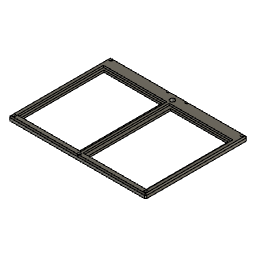
SensorBox-Zanzibar_Waterproofing v12 (Autodesk Fusion 360 design; units mm, degrees)
Autodesk Fusion 360 part; units mm, degrees
note: some values were not read from the file. Set by a fixed rule: which face or edge a step refers to.
sketch "Sketch1" plane through (0, 0, 0) normal (0, 0, 1) x (1, 0, 0) in component "Panel_Top"
  line L0 (27.5294, 43.3117) -> (202.5294, 43.3117)
  line L1 (202.5294, 43.3117) -> (202.5294, 173.3117)
  line L2 (202.5294, 173.3117) -> (27.5294, 173.3117)
  line L3 (27.5294, 173.3117) -> (27.5294, 43.3117)
  line L4 (197.5294, 159.5617) -> (32.5294, 159.5617)
  line L5 (32.5294, 159.5617) -> (32.5294, 49.5617)
  line L6 (32.5294, 49.5617) -> (197.5294, 49.5617)
  line L7 (197.5294, 49.5617) -> (197.5294, 159.5617)
  line L8 (197.5294, 159.5617) -> (32.5294, 49.5617) construction
  line L9 (32.5294, 159.5617) -> (197.5294, 49.5617) construction
  line L10 (116.5294, 159.5617) -> (113.5294, 159.5617)
  line L11 (113.5294, 159.5617) -> (113.5294, 49.5617)
  line L12 (113.5294, 49.5617) -> (116.5294, 49.5617)
  line L13 (116.5294, 49.5617) -> (116.5294, 159.5617)
  line L14 (116.5294, 159.5617) -> (113.5294, 49.5617) construction
  line L15 (113.5294, 159.5617) -> (116.5294, 49.5617) construction
  line L16 (27.5294, 108.3117) -> (32.5294, 104.5617)
  line L17 (115.0294, 43.3117) -> (115.0294, 49.5617)
  line L18 (109.5294, 157.0617) -> (35.5294, 157.0617)
  line L19 (35.5294, 157.0617) -> (35.5294, 52.0617)
  line L20 (35.5294, 52.0617) -> (109.5294, 52.0617)
  line L21 (109.5294, 52.0617) -> (109.5294, 157.0617)
  line L22 (120.5294, 157.0617) -> (194.5294, 157.0617)
  line L23 (194.5294, 157.0617) -> (194.5294, 52.0617)
  line L24 (194.5294, 52.0617) -> (120.5294, 52.0617)
  line L25 (120.5294, 52.0617) -> (120.5294, 157.0617)
  circle A0 centre (115, 165) radius 3
  circle A1 centre (30.9, 47.1432) radius 1
  line L26 (115.0294, 120.0286) -> (115.0294, 79)
  circle A2 centre (199.1589, 47.1432) radius 1
  circle A3 centre (31.1445, 170.3984) radius 1
  circle A4 centre (198.9143, 170.3984) radius 1
  circle A5 centre (115.0294, 46.0617) radius 1
  line L27 (115.0294, 45.0617) -> (115.0294, 43.3117)
  line L28 (115.0294, 45.0617) -> (115.0294, 43.3117)
  circle A6 centre (31.1445, 170.3984) radius 2
  circle A7 centre (30.9, 47.1432) radius 2
  circle A8 centre (115.0294, 46.0617) radius 2
  circle A9 centre (199.1589, 47.1432) radius 2
  circle A10 centre (198.9143, 170.3984) radius 2
  circle A11 centre (103.0229, 171.842) radius 1
  circle A12 centre (127.025, 171.7921) radius 1
  circle A13 centre (103.0229, 171.842) radius 2
  circle A14 centre (127.025, 171.7921) radius 2
  point P0 (115.0294, 104.5617)
  point P1 (115.0294, 104.5617)
  point P2 (73.0294, 104.5617)
  point P3 (115, 165)
  point P4 (103.0229, 171.842)
  dimension "d29" = 175
  dimension "d30" = 130
  dimension "d31" = 165
  dimension "d32" = 110
  dimension "d33" = 3
  dimension "d34" = 81
  dimension "d35" = 81
  dimension "d36" = 74
  dimension "d37" = 105
  dimension "d38" = 74
  dimension "d39" = 105
  dimension "d47" = 6
  dimension "d85" = 2
  dimension "d86" = 2
  dimension "d89" = 2
  dimension "d90" = 2
  dimension "d92" = 2
  dimension "d93" = 1.75
  dimension "d213" = 4
  dimension "d214" = 4
  dimension "d215" = 4
  dimension "d216" = 4
  dimension "d217" = 4
  dimension "d223" = 2
  dimension "d224" = 2
  dimension "d225" = 4
  dimension "d226" = 4
  constraint horizontal L0
  constraint vertical L1
  constraint horizontal L2
  constraint vertical L3
  constraint horizontal L4
  constraint perpendicular L4 L5
  constraint parallel L4 L6
  constraint parallel L5 L7
  constraint coincident L8 P1
  constraint coincident L9 P1
  constraint horizontal L10
  constraint perpendicular L10 L11
  constraint parallel L10 L12
  constraint parallel L11 L13
  constraint coincident L14 P1
  constraint coincident L15 P1
  constraint coincident P1 P0
  constraint midpoint L3 L16.start
  constraint midpoint L5 L16.end
  constraint midpoint L0 L17.start
  constraint midpoint L6 L17.end
  constraint perpendicular L6 L17
  constraint equal L16 L17
  constraint horizontal L18
  constraint perpendicular L18 L19
  constraint parallel L18 L20
  constraint parallel L19 L21
  constraint perpendicular L22 L23
  constraint parallel L22 L24
  constraint parallel L23 L25
  constraint parallel L25 L26
  constraint coincident L17 A5.centre
  constraint coincident A5 L27.start
  constraint coincident L17 L27.start
  constraint perpendicular L0 L27
  constraint coincident P3 A0.centre
  constraint concentric A3 A6
  constraint concentric A1 A7
  constraint concentric A5 A8
  constraint concentric A2 A9
  constraint concentric A4 A10
  constraint coincident P4 A11.centre
  constraint concentric A11 A13
  constraint concentric A12 A14
  measures "d29" distance of L0.start L0.end
  measures "d30" distance of L0.start L2.end
  measures "d31" distance of L5.end L6.end
  measures "d32" distance of L4.end L5.end
  measures "d33" distance of L11.end L12.end
  measures "d34" distance of L5.end L11.end
  measures "d35" distance of L6.end L12.end
  measures "d36" distance of L19.end L20.end
  measures "d37" distance of L18.end L19.end
  measures "d38" distance of L23.end L24.end
  measures "d39" distance of L22.end L23.end
  measures "d47" diameter of A0
  measures "d85" diameter of A1
  measures "d86" diameter of A2
  measures "d89" diameter of A3
  measures "d90" diameter of A4
  measures "d92" diameter of A5
  measures "d93" distance of L17.start L27.start
  measures "d213" diameter of A6
  measures "d214" diameter of A7
  measures "d215" diameter of A8
  measures "d216" diameter of A9
  measures "d217" diameter of A10
  measures "d223" diameter of A11
  measures "d224" diameter of A12
  measures "d225" diameter of A13
  measures "d226" diameter of A14
extrude "Extrude2" add sketch "Sketch1" along normal blind 5 contours L0 L3 L5 L6 L12 L16 L17 L27 L28 A8 | L0 L1 L2 L3 L4 L5 L6 L7 L10 L12 L16 L17 L27 L28 A8 A13 A14 | L17 A5 L27 L28 A8 | L17 A5 L27 L28 A8 | L17 A5 | L17 A5 | L2 A13 | L2 A14 | L4 L6 L10 L11 L12 L13 | A0 | A1 | A2 | A3 | A4 | A6 | A7 | A9 | A10 | A11 | A12 picked at (103.0478, 173.1542) picked at (127.0499, 173.1375) makes body 1 in component "Panel_Top"
extrude "Extrude3" add sketch "Sketch1" along normal blind 2.5 contours L4 L5 L6 L11 | L4 L6 L7 L13 bodies 1 in component "Panel_Top"
chamfer "Chamfer1" distance 1.5 angle 45 8 edges at (115.0294, 173.3117, 5) (115.0294, 43.3117, 5) (202.5294, 108.3117, 5) (202.5294, 43.3117, 2.5) (202.5294, 173.3117, 2.5) (27.5294, 173.3117, 2.5) (27.5294, 108.3117, 5) (27.5294, 43.3117, 2.5) on bodies 1 in component "Panel_Top"
extrude "Extrude4" cut sketch "Sketch1" along normal blind 10 contours A0 bodies 1 in component "Panel_Top"
sketch "Sketch1 (2)" plane through (0, 0, 0) normal (0, 0, 1) x (1, 0, 0) in component "Box"
  line L0 (200.9294, 173.7581) -> (25.9294, 173.7581)
  line L1 (200.9294, 43.7581) -> (200.9294, 173.7581)
  line L2 (25.9294, 43.7581) -> (200.9294, 43.7581)
  line L3 (25.9294, 173.7581) -> (25.9294, 43.7581)
  line L4 (100.1921, 43.7581) -> (100.1921, 49.5617)
  line L5 (76.1646, 173.7581) -> (76.1646, 167.0617)
  line L6 (100.1292, 173.7581) -> (100.1292, 167.0617)
  line L7 (195.9294, 170.3581) -> (30.9294, 170.3581)
  line L8 (30.9294, 170.3581) -> (30.9294, 50.3581)
  line L9 (30.9294, 50.3581) -> (195.9294, 50.3581)
  line L10 (195.9294, 50.3581) -> (195.9294, 170.3581)
  line L11 (195.9294, 170.3581) -> (30.9294, 50.3581) construction
  line L12 (30.9294, 170.3581) -> (195.9294, 50.3581) construction
  circle A0 centre (29.5445, 170.3984) radius 1
  line L13 (25.9294, 173.7581) -> (30.9294, 170.3581)
  circle A1 centre (197.5001, 170.373) radius 1
  circle A2 centre (29.3, 47.1432) radius 1
  circle A3 centre (197.5001, 47.1432) radius 1
  circle A4 centre (113.425, 46.5081) radius 1
  line L14 (113.4294, 43.7581) -> (113.4294, 45.5081)
  line L15 (35.5295, 157.0617) -> (191.3258, 157.0617)
  line L16 (191.3258, 157.0617) -> (191.3258, 52.0619)
  line L17 (191.3258, 52.0619) -> (35.5295, 52.0619)
  line L18 (35.5295, 52.0619) -> (35.5295, 157.0617)
  line L19 (99.995, 157.0617) -> (129.995, 157.0617)
  line L20 (129.995, 157.0617) -> (129.995, 169.1149)
  line L21 (129.995, 169.1149) -> (99.995, 169.1149)
  line L22 (99.995, 169.1149) -> (99.995, 157.0617)
  line L23 (35.5295, 135.5381) -> (30.9294, 135.3581)
  line L24 (65.9281, 157.0617) -> (65.9281, 170.6598)
  line L25 (162.4706, 157.0617) -> (162.4706, 168.7581)
  line L26 (191.3258, 133.7581) -> (195.9294, 133.7581)
  line L27 (35.5295, 83.7581) -> (30.9294, 83.7581)
  line L28 (191.3258, 83.7581) -> (195.9294, 83.7581)
  line L29 (67.5294, 52.0619) -> (67.5294, 50.3581)
  line L30 (162.4706, 52.0619) -> (162.4706, 50.3581)
  line L31 (50, 162) -> (80, 162)
  line L32 (80, 162) -> (80, 157)
  line L33 (80, 157) -> (50, 157)
  line L34 (50, 157) -> (50, 162)
  line L35 (180, 162) -> (150, 162)
  line L36 (180, 157) -> (180, 162)
  line L37 (150, 157) -> (180, 157)
  line L38 (150, 162) -> (150, 157)
  line L39 (25.9294, 99.9709) -> (30.9294, 99.9709)
  line L40 (195.9294, 99.9709) -> (200.9294, 99.9709)
  line L41 (159.383, 124.881) -> (70.383, 124.881)
  line L42 (70.383, 124.881) -> (70.383, 150.281)
  line L43 (70.383, 150.281) -> (159.383, 150.281)
  line L44 (159.383, 150.281) -> (159.383, 124.881)
  line L45 (159.383, 124.881) -> (70.383, 150.281) construction
  line L46 (70.383, 124.881) -> (159.383, 150.281) construction
  line L47 (94.9348, 114.6136) -> (54.9348, 114.6136)
  line L48 (54.9348, 114.6136) -> (54.9348, 61.6136)
  line L49 (54.9348, 61.6136) -> (94.9348, 61.6136)
  line L50 (94.9348, 61.6136) -> (94.9348, 114.6136)
  line L51 (94.9348, 114.6136) -> (54.9348, 61.6136) construction
  line L52 (54.9348, 114.6136) -> (94.9348, 61.6136) construction
  line L53 (54.9348, 114.6136) -> (64.9348, 114.6136)
  line L54 (64.9348, 114.6136) -> (64.9348, 104.6136)
  line L55 (64.9348, 104.6136) -> (54.9348, 104.6136)
  line L56 (54.9348, 104.6136) -> (54.9348, 114.6136)
  line L57 (54.9348, 61.6136) -> (64.9348, 61.6136)
  line L58 (64.9348, 61.6136) -> (64.9348, 71.6136)
  line L59 (64.9348, 71.6136) -> (54.9348, 71.6136)
  line L60 (54.9348, 71.6136) -> (54.9348, 61.6136)
  line L61 (94.9348, 114.6136) -> (84.9348, 114.6136)
  line L62 (84.9348, 114.6136) -> (84.9348, 104.6136)
  line L63 (84.9348, 104.6136) -> (94.9348, 104.6136)
  line L64 (94.9348, 104.6136) -> (94.9348, 114.6136)
  line L65 (94.9348, 61.6136) -> (84.9348, 61.6136)
  line L66 (84.9348, 61.6136) -> (84.9348, 71.6136)
  line L67 (84.9348, 71.6136) -> (94.9348, 71.6136)
  line L68 (94.9348, 71.6136) -> (94.9348, 61.6136)
  line L69 (64.9348, 104.6136) -> (51.9348, 104.6136)
  line L70 (51.9348, 104.6136) -> (51.9348, 117.6136)
  line L71 (51.9348, 117.6136) -> (64.9348, 117.6136)
  line L72 (64.9348, 117.6136) -> (64.9348, 104.6136)
  line L73 (64.9348, 71.6136) -> (51.9348, 71.6136)
  line L74 (51.9348, 71.6136) -> (51.9348, 58.6136)
  line L75 (51.9348, 58.6136) -> (64.9348, 58.6136)
  line L76 (64.9348, 58.6136) -> (64.9348, 71.6136)
  line L77 (84.9348, 71.6136) -> (97.9348, 71.6136)
  line L78 (97.9348, 71.6136) -> (97.9348, 58.6136)
  line L79 (97.9348, 58.6136) -> (84.9348, 58.6136)
  line L80 (84.9348, 58.6136) -> (84.9348, 71.6136)
  line L81 (84.9348, 104.6136) -> (97.9348, 104.6136)
  line L82 (97.9348, 104.6136) -> (97.9348, 117.6136)
  line L83 (97.9348, 117.6136) -> (84.9348, 117.6136)
  line L84 (84.9348, 117.6136) -> (84.9348, 104.6136)
  line L85 (159.2809, 101.4464) -> (104.2809, 101.4464)
  line L86 (104.2809, 101.4464) -> (104.2809, 76.4464)
  line L87 (104.2809, 76.4464) -> (159.2809, 76.4464)
  line L88 (159.2809, 76.4464) -> (159.2809, 101.4464)
  line L89 (159.2809, 101.4464) -> (104.2809, 76.4464) construction
  line L90 (104.2809, 101.4464) -> (159.2809, 76.4464) construction
  circle A5 centre (104.2809, 101.4464) radius 1.25
  circle A6 centre (104.2809, 76.4464) radius 1.25
  circle A7 centre (159.2809, 101.4464) radius 1.25
  circle A8 centre (159.2809, 76.4464) radius 1.25
  circle A9 centre (70.383, 150.281) radius 1.6
  circle A10 centre (70.383, 124.881) radius 1.6
  circle A11 centre (159.383, 150.281) radius 1.6
  circle A12 centre (159.383, 124.881) radius 1.6
  line L91 (30.9294, 116.2794) -> (35.5295, 116.2794)
  line L92 (35.5295, 116.2794) -> (35.5295, 101.2775)
  line L93 (35.5295, 101.2775) -> (30.9294, 101.2775)
  line L94 (30.9294, 101.2775) -> (30.9294, 116.2794)
  line L95 (191.3258, 101.2799) -> (195.9294, 101.2799)
  line L96 (195.9294, 101.2799) -> (195.9294, 116.2759)
  line L97 (195.9294, 116.2759) -> (191.3258, 116.2759)
  line L98 (191.3258, 116.2759) -> (191.3258, 101.2799)
  circle A13 centre (104.2809, 101.4464) radius 2.25
  circle A14 centre (104.2809, 76.4464) radius 2.25
  circle A15 centre (159.2809, 101.4464) radius 2.25
  circle A16 centre (159.2809, 76.4464) radius 2.25
  circle A17 centre (127.0246, 171.7917) radius 1
  line L99 (114.995, 172.8091) -> (114.995, 171)
  circle A18 centre (103.0221, 171.8383) radius 1
  point P0 (113.4294, 110.3581)
  point P1 (113.4294, 110.3581)
  point P2 (114.883, 137.581)
  point P3 (74.9348, 88.1136)
  point P4 (113.4294, 110.3581)
  point P5 (131.7809, 88.9464)
  dimension "d50" = 175
  dimension "d51" = 130
  dimension "d68" = 5.8036
  dimension "d69" = 165
  dimension "d70" = 120
  dimension "d77" = 2
  dimension "d82" = 2
  dimension "d83" = 2
  dimension "d84" = 2
  dimension "d94" = 2
  dimension "d95" = 1.75
  dimension "d120" = 30
  dimension "d127" = 35
  dimension "d128" = 35
  dimension "d146" = 89
  dimension "d147" = 25.4
  dimension "d155" = 40
  dimension "d156" = 53
  dimension "d157" = 10
  dimension "d158" = 10
  dimension "d159" = 10
  dimension "d160" = 10
  dimension "d161" = 10
  dimension "d162" = 10
  dimension "d163" = 10
  dimension "d164" = 10
  dimension "d165" = 13
  dimension "d166" = 13
  dimension "d167" = 13
  dimension "d168" = 13
  dimension "d169" = 13
  dimension "d170" = 13
  dimension "d171" = 13
  dimension "d172" = 13
  dimension "d175" = 55
  dimension "d176" = 25
  dimension "d177" = 2.5
  dimension "d178" = 2.5
  dimension "d179" = 2.5
  dimension "d180" = 2.5
  dimension "d181" = 3.2
  dimension "d182" = 3.2
  dimension "d183" = 3.2
  dimension "d184" = 3.2
  dimension "d207" = 4.5
  dimension "d208" = 4.5
  dimension "d209" = 4.5
  dimension "d210" = 4.5
  dimension "d221" = 2
  dimension "d222" = 2
  constraint horizontal L2
  constraint vertical L1
  constraint horizontal L0
  constraint vertical L3
  constraint coincident L2 L4.start
  constraint coincident L0 L5.start
  constraint coincident L0 L6.start
  constraint horizontal L7
  constraint perpendicular L7 L8
  constraint parallel L7 L9
  constraint parallel L8 L10
  constraint coincident L11 P4
  constraint coincident L12 P4
  constraint midpoint L2 L14.start
  constraint coincident A4 L14.end
  constraint perpendicular L2 L14
  constraint horizontal L15
  constraint vertical L16
  constraint horizontal L17
  constraint vertical L18
  constraint horizontal L19
  constraint vertical L20
  constraint horizontal L21
  constraint vertical L22
  constraint coincident L15 L19.start
  constraint coincident L8 L23.end
  constraint coincident L18 L23.start
  constraint coincident L15 L24.start
  constraint perpendicular L7 L24
  constraint coincident L10 L28.end
  constraint perpendicular L10 L28
  constraint coincident L16 L28.start
  constraint coincident L10 L26.end
  constraint perpendicular L10 L26
  constraint coincident L16 L26.start
  constraint coincident L17 L29.start
  constraint coincident L9 L29.end
  constraint perpendicular L9 L29
  constraint coincident L17 L30.start
  constraint coincident L9 L30.end
  constraint perpendicular L9 L30
  constraint horizontal L31
  constraint vertical L32
  constraint horizontal L33
  constraint vertical L34
  constraint coincident P4 P1
  constraint equal L23 L26
  constraint coincident L8 L27.end
  constraint perpendicular L8 L27
  constraint coincident L3 L39.start
  constraint coincident L8 L39.end
  constraint perpendicular L8 L39
  constraint coincident L10 L40.start
  constraint coincident L1 L40.end
  constraint perpendicular L1 L40
  constraint equal L39 L40
  constraint horizontal L41
  constraint perpendicular L41 L42
  constraint parallel L41 L43
  constraint parallel L42 L44
  constraint coincident L45 P2
  constraint coincident L46 P2
  constraint horizontal L47
  constraint perpendicular L47 L48
  constraint parallel L47 L49
  constraint parallel L48 L50
  constraint coincident L51 P3
  constraint coincident L52 P3
  constraint horizontal L53
  constraint vertical L54
  constraint horizontal L55
  constraint vertical L56
  constraint horizontal L57
  constraint vertical L58
  constraint horizontal L59
  constraint vertical L60
  constraint horizontal L61
  constraint vertical L62
  constraint horizontal L63
  constraint vertical L64
  constraint horizontal L65
  constraint vertical L66
  constraint horizontal L67
  constraint vertical L68
  constraint horizontal L69
  constraint vertical L70
  constraint horizontal L71
  constraint vertical L72
  constraint horizontal L73
  constraint vertical L74
  constraint horizontal L75
  constraint vertical L76
  constraint horizontal L77
  constraint vertical L78
  constraint horizontal L79
  constraint vertical L80
  constraint horizontal L81
  constraint vertical L82
  constraint horizontal L83
  constraint vertical L84
  constraint horizontal L85
  constraint perpendicular L85 L86
  constraint parallel L85 L87
  constraint parallel L86 L88
  constraint coincident L89 P5
  constraint coincident L90 P5
  constraint coincident L85.end L86.start
  constraint coincident L86.end L87.start
  constraint coincident L85.start L88.end
  constraint coincident L87.end L88.start
  constraint coincident L42.end L43.start
  constraint coincident L41.end L42.start
  constraint coincident L43.end L44.start
  constraint coincident L41.start L44.end
  constraint horizontal L91
  constraint vertical L92
  constraint horizontal L93
  constraint vertical L94
  constraint coincident L18 L92.end
  constraint coincident L8 L91.start
  constraint horizontal L95
  constraint vertical L96
  constraint horizontal L97
  constraint vertical L98
  constraint coincident L10 L96.end
  constraint coincident L16 L95.start
  constraint concentric A5 A13
  constraint concentric A6 A14
  constraint concentric A7 A15
  constraint concentric A8 A16
  constraint perpendicular L7 L99
  measures "d50" distance of L1.start L2.start
  measures "d51" distance of L0.end L2.start
  measures "d68" distance of L4.start L4.end
  measures "d69" distance of L8.end L9.end
  measures "d70" distance of L7.end L8.end
  measures "d77" diameter of A0
  measures "d82" diameter of A1
  measures "d83" diameter of A2
  measures "d84" diameter of A3
  measures "d94" diameter of A4
  measures "d95" distance of L14.start L14.end
  measures "d120" distance of L19.start L19.end
  measures "d127" distance of L7.end L23.end
  measures "d128" distance of L7.end L24.end
  measures "d146" distance of L42.end L43.end
  measures "d147" distance of L41.end L42.end
  measures "d155" distance of L48.end L49.end
  measures "d156" distance of L47.end L48.end
  measures "d157" distance of L47.end L53.end
  measures "d158" distance of L47.end L55.end
  measures "d159" distance of L48.end L57.end
  measures "d160" distance of L48.end L59.end
  measures "d161" distance of L47.start L61.end
  measures "d162" distance of L47.start L63.end
  measures "d163" distance of L49.end L65.end
  measures "d164" distance of L49.end L67.end
  measures "d165" distance of L54.end L69.end
  measures "d166" distance of L54.end L71.end
  measures "d167" distance of L58.end L73.end
  measures "d168" distance of L58.end L75.end
  measures "d169" distance of L66.end L77.end
  measures "d170" distance of L66.end L79.end
  measures "d171" distance of L62.end L81.end
  measures "d172" distance of L62.end L83.end
  measures "d175" distance of L86.end L87.end
  measures "d176" distance of L85.end L86.end
  measures "d177" diameter of A5
  measures "d178" diameter of A6
  measures "d179" diameter of A7
  measures "d180" diameter of A8
  measures "d181" diameter of A9
  measures "d182" diameter of A10
  measures "d183" diameter of A11
  measures "d184" diameter of A12
  measures "d207" diameter of A13
  measures "d208" diameter of A14
  measures "d209" diameter of A15
  measures "d210" diameter of A16
  measures "d221" diameter of A17
  measures "d222" diameter of A18
extrude "Extrude5" cut sketch "Sketch1" along normal blind 10 contours L17 A5 | L17 A5 | A1 | A2 | A3 | A4 | A11 | A12 bodies 1 in component "Panel_Top"
extrude "Extrude5'" add sketch "Sketch1 (2)" along normal blind 5 separate body contours L0 L1 L6 L7 L10 L40 L96 | L0 L5 L6 L7 | L1 L2 L3 L8 L9 L10 L39 L40 | L0 L5 L7 A0 L13 | L6 L7 L10 L15 L16 L20 L21 L26 L35 L36 L38 | L6 L7 L15 L21 L22 L24 L31 L32 | L10 L16 L28 L95 | L3 L8 A0 L13 L39 L94 | L15 L19 L20 L21 L22 | L9 L10 L16 L17 L28 L30 | L10 L16 L95 L96 L97 L98 | A0 L13 | A0 L13 | L7 L8 L15 L18 L23 L24 L31 L34 | L10 L16 L26 L97 | L15 L16 L17 L18 L19 L32 L33 L34 L36 L37 L38 L92 L98 | L8 L18 L27 L93 | L15 L24 L31 L32 | L15 L24 L31 L34 | L9 L17 L29 L30 | L8 L18 L91 L92 L93 L94 | L8 L9 L17 L18 L27 L29 | L8 L18 L23 L91 | L15 L32 L33 L34 | L15 L25 L35 L38 | L15 L36 L37 L38 | L15 L25 L35 L36 | A1 | A2 | A3 | A4 | L41 L42 A10 | L41 L42 L43 L44 A9 A10 A11 A12 | L41 L42 A10 | L41 L44 A12 | L41 L44 A12 | L42 L43 A9 | L42 L43 A9 | L43 L44 A11 | L43 L44 A11 | L47 L50 L61 L62 L63 L64 L81 L84 | L47 L50 L61 L64 L81 L82 L83 L84 | L47 L48 L49 L50 L54 L55 L58 L59 L62 L63 L66 L67 L69 L72 L73 L76 L77 L80 L81 L84 | L47 L48 L53 L54 L55 L56 L69 L72 | L47 L48 L53 L56 L69 L70 L71 L72 | L49 L50 L65 L68 L77 L78 L79 L80 | L49 L50 L65 L66 L67 L68 L77 L80 | L48 L49 L57 L58 L59 L60 L73 L76 | L48 L49 L57 L60 L73 L74 L75 L76 | L85 L86 A5 A13 | L85 L86 A5 A13 | L85 L86 L87 L88 A13 A14 A15 A16 | L85 L86 A5 | L85 L86 A5 | L85 L88 A7 A15 | L85 L88 A7 A15 | L85 L88 A7 | L85 L88 A7 | L86 L87 A6 A14 | L86 L87 A6 A14 | L87 L88 A8 A16 | L87 L88 A8 A16 | L86 L87 A6 | L86 L87 A6 | L87 L88 A8 | L87 L88 A8 | A17 | A18 makes body 2 in component "Box"
extrude "Extrude6" add sketch "Sketch1 (2)" along normal blind 35 from surface at 5 contours L0 L1 L6 L7 L10 L40 L96 | L0 L5 L6 L7 | L1 L2 L3 L8 L9 L10 L39 L40 | L0 L5 L7 A0 L13 | L3 L8 A0 L13 L39 L94 | A0 L13 | A0 L13 | A1 | A2 | A3 | A4 | A17 | A18 bodies 2 in component "Box"
chamfer "Chamfer3" distance 1.5 angle 45 8 edges at (25.9294, 43.7581, 20) (113.4294, 43.7581, 0) (25.9294, 108.7581, 0) (200.9294, 108.7581, 0) (113.4294, 173.7581, 0) (200.9294, 43.7581, 20) (200.9294, 173.7581, 20) (25.9294, 173.7581, 20) on bodies 2 in component "Box"
extrude "Extrude6'" add sketch "Sketch1" along normal blind 5 contours A0 bodies 1 in component "Panel_Top"
extrude "Extrude7" cut sketch "Sketch1" along normal blind 5 contours A0 bodies 1 in component "Panel_Top"
sketch "Sketch2" plane through (0, 0, 0) normal (1, 0, 0) x (0, 1, 0) in component "Box"
  line L0 (173.7584, 40) -> (43.75, 40)
  line L1 (43.75, 40) -> (43.75, 0)
  line L2 (43.75, 0) -> (173.7584, 0)
  line L3 (173.7584, 0) -> (173.7584, 40)
  line L4 (101.2542, 40) -> (116.2542, 40)
  line L5 (116.2542, 0) -> (101.2542, 0)
  line L6 (116.2929, 10.1303) -> (101.2929, 10.1303)
  line L7 (101.2929, 10.1303) -> (101.2929, 5.1303)
  line L8 (101.2929, 5.1303) -> (116.2929, 5.1303)
  line L9 (116.2929, 5.1303) -> (116.2929, 10.1303)
  line L10 (116.2929, 10.1303) -> (101.2929, 5.1303) construction
  line L11 (101.2929, 10.1303) -> (116.2929, 5.1303) construction
  point P0 (108.7929, 7.6303)
  point P1 (108.7929, 7.6303)
  dimension "d104" = 15
  dimension "d105" = 15
  dimension "d106" = 5
  constraint horizontal L0
  constraint vertical L1
  constraint horizontal L2
  constraint vertical L3
  constraint horizontal L4
  constraint parallel L4 L5
  constraint horizontal L6
  constraint perpendicular L6 L7
  constraint parallel L6 L8
  constraint parallel L7 L9
  constraint coincident L10 P1
  constraint coincident L11 P1
  constraint coincident P1 P0
  measures "d104" distance of L5.start L5.end
  measures "d105" distance of L7.end L8.end
  measures "d106" distance of L6.end L7.end
extrude "Extrude7'" cut sketch "Sketch2" along normal blind 300 contours L6 L7 L8 L9 bodies 2 in component "Box"
sketch "Sketch3" plane through (0, 0, 0) normal (0, 1, 0) x (1, 0, 0) in component "Box"
  line L0 (197.53, -35) -> (202.5, -35)
  line L1 (202.5, -35) -> (202.5, -5)
  line L2 (202.5, -5) -> (197.53, -5)
  line L3 (197.53, -5) -> (197.53, -35)
  line L4 (200.9998, -35) -> (205.0157, -17.4537)
  line L5 (205.0157, -17.4537) -> (206.4412, -17.78)
  line L6 (206.4412, -17.78) -> (202.4253, -35.3263)
  line L7 (202.4253, -35.3263) -> (200.9998, -35)
  line L8 (202.4253, -23.3263) -> (200.9998, -23)
  line L9 (200.9998, -23) -> (205.0157, -5.4537)
  line L10 (206.4412, -5.78) -> (202.4253, -23.3263)
  line L11 (205.0157, -5.4537) -> (206.4412, -5.78)
  line L12 (27.5294, -40) -> (202.5325, -40)
  line L13 (202.5325, -40) -> (202.5325, 0)
  line L14 (202.5325, 0) -> (27.5294, 0)
  line L15 (27.5294, 0) -> (27.5294, -40)
  line L16 (115.0309, -35.0662) -> (115.0309, -10)
  line L17 (27.6366, -35.3263) -> (29.0621, -35)
  line L18 (29.0621, -35) -> (25.0462, -17.4537)
  line L19 (23.6207, -17.78) -> (27.6366, -35.3263)
  line L20 (25.0462, -17.4537) -> (23.6207, -17.78)
  line L21 (27.6366, -23.3263) -> (29.0621, -23)
  line L22 (29.0621, -23) -> (25.0462, -5.4537)
  line L23 (23.6207, -5.78) -> (27.6366, -23.3263)
  line L24 (25.0462, -5.4537) -> (23.6207, -5.78)
  dimension "d110" = 18
  dimension "d111" = 18
  dimension "d115" = 18
  dimension "d116" = 18
  constraint horizontal L0
  constraint vertical L1
  constraint horizontal L2
  constraint vertical L3
  constraint perpendicular L4 L5
  constraint parallel L4 L6
  constraint parallel L5 L7
  constraint coincident L0 L4.start
  constraint perpendicular L9 L11
  constraint parallel L9 L10
  constraint parallel L8 L11
  constraint horizontal L12
  constraint vertical L13
  constraint horizontal L14
  constraint vertical L15
  constraint perpendicular L12 L16
  constraint perpendicular L18 L20
  constraint parallel L18 L19
  constraint parallel L17 L20
  constraint perpendicular L22 L24
  constraint parallel L22 L23
  constraint parallel L21 L24
  measures "d110" distance of L4.start L4.end
  measures "d111" distance of L8.end L9.end
  measures "d115" distance of L17.end L18.end
  measures "d116" distance of L22.end L21.end
extrude "Extrude10" add sketch "Sketch1 (2)" along normal blind 2 from surface at 5 contours L15 L19 L20 L21 L22 | L15 L16 L17 L18 L19 L32 L33 L34 L36 L37 L38 L92 L98 | L15 L32 L33 L34 | L15 L36 L37 L38 | L41 L42 A10 | L41 L42 L43 L44 A9 A10 A11 A12 | L41 L42 A10 | L41 L44 A12 | L41 L44 A12 | L42 L43 A9 | L42 L43 A9 | L43 L44 A11 | L43 L44 A11 | L47 L50 L61 L62 L63 L64 L81 L84 | L47 L50 L61 L64 L81 L82 L83 L84 | L47 L48 L49 L50 L54 L55 L58 L59 L62 L63 L66 L67 L69 L72 L73 L76 L77 L80 L81 L84 | L47 L48 L53 L54 L55 L56 L69 L72 | L47 L48 L53 L56 L69 L70 L71 L72 | L49 L50 L65 L68 L77 L78 L79 L80 | L49 L50 L65 L66 L67 L68 L77 L80 | L48 L49 L57 L58 L59 L60 L73 L76 | L48 L49 L57 L60 L73 L74 L75 L76 | L85 L86 A5 A13 | L85 L86 A5 A13 | L85 L86 L87 L88 A13 A14 A15 A16 | L85 L86 A5 | L85 L86 A5 | L85 L88 A7 A15 | L85 L88 A7 A15 | L85 L88 A7 | L85 L88 A7 | L86 L87 A6 A14 | L86 L87 A6 A14 | L87 L88 A8 A16 | L87 L88 A8 A16 | L86 L87 A6 | L86 L87 A6 | L87 L88 A8 | L87 L88 A8 bodies 2 in component "Box"
extrude "Extrude11" cut sketch "Sketch1 (2)" against normal blind 7 from surface at 40 contours A0 L13 | A0 L13 | A1 | A2 | A3 | A4 | A17 | A18 bodies 2 in component "Box"
extrude "Extrude13" cut sketch "Sketch1 (2)" along normal blind 7 contours L15 L24 L31 L32 | L15 L24 L31 L34 | L15 L32 L33 L34 | L15 L25 L35 L38 | L15 L36 L37 L38 | L15 L25 L35 L36 bodies 2 in component "Box"
extrude "Extrude15" add sketch "Sketch1 (2)" along normal blind 4 from surface at 7 contours L41 L42 A10 | L41 L42 A10 | L41 L44 A12 | L41 L44 A12 | L42 L43 A9 | L42 L43 A9 | L43 L44 A11 | L43 L44 A11 bodies 2 in component "Box"
extrude "Extrude17" add sketch "Sketch1 (2)" along normal blind 7 from surface at 7 contours L47 L50 L61 L64 L81 L82 L83 L84 | L47 L48 L53 L56 L69 L70 L71 L72 | L49 L50 L65 L68 L77 L78 L79 L80 | L48 L49 L57 L60 L73 L74 L75 L76 bodies 2 in component "Box"
extrude "Extrude18" cut sketch "Sketch1 (2)" along normal blind 5 contours L8 L18 L91 L92 L93 L94 bodies 2 in component "Box"
extrude "Extrude19" cut sketch "Sketch1 (2)" along normal blind 5 contours L10 L16 L95 L96 L97 L98 bodies 2 in component "Box"
extrude "Extrude21" cut sketch "Sketch1 (2)" along normal blind 10 contours L85 L86 A5 | L85 L86 A5 | L85 L88 A7 | L85 L88 A7 | L86 L87 A6 | L86 L87 A6 | L87 L88 A8 | L87 L88 A8 bodies 2 in component "Box"
extrude "Extrude22" cut sketch "Sketch1 (2)" along normal blind 2 contours L85 L86 A5 A13 | L85 L86 A5 A13 | L85 L86 A5 | L85 L86 A5 | L85 L88 A7 A15 | L85 L88 A7 A15 | L85 L88 A7 | L85 L88 A7 | L86 L87 A6 A14 | L86 L87 A6 A14 | L87 L88 A8 A16 | L87 L88 A8 A16 | L86 L87 A6 | L86 L87 A6 | L87 L88 A8 | L87 L88 A8 bodies 2 in component "Box"
extrude "Extrude8" cut sketch "Sketch1" against normal blind 2 from surface at 5 contours L17 A5 L27 L28 A8 | L17 A5 L27 L28 A8 | L17 A5 | L17 A5 | L2 A13 | L2 A13 | L2 A14 | L2 A14 | A1 | A2 | A3 | A4 | A6 | A7 | A9 | A10 | A11 | A12 bodies 1 in component "Panel_Top"
component "Panel_Top" placed x (1, 0, 0) y (0, 1, 0) z (0, 0, 1) at (0, 0, 0)
component "Box" placed x (1, 0, 0) y (0, 1, 0) z (0, 0, 1) at (0, 0, 0)
